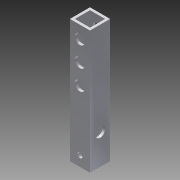
# Autodesk Inventor part: 1x1 vertical
Saved by Autodesk Inventor 2015 (Build 190159000, 159)
## iProperties
Created: 2015-01-27
Part Number: 1x1 vertical
Material: Aluminum 6061
Document SubType Name: Modeling
Designer: Admin
Density: 2.7 g/cm^3
Appearance: Aluminum - Flat
Author: Admin
Autodesk Inventor part; units mm, degrees
ref_plane "YZ Plane" through (0, 0, 0) normal (1, 0, 0) x (0, 1, 0)
ref_plane "XZ Plane" through (0, 0, 0) normal (0, 1, 0) x (-1, 0, 0)
ref_plane "XY Plane" through (0, 0, 0) normal (0, 0, 1) x (1, 0, 0)
sketch "Sketch1" plane through (0, 0, 0) normal (0, 1, 0) x (-1, 0, 0)
  line L0 (0, 0) -> (-25.4, 0)
  line L1 (-25.4, 0) -> (-25.4, -25.4)
  line L2 (-25.4, -25.4) -> (0, -25.4)
  line L3 (0, -25.4) -> (0, 0)
  line L4 (-3.175, -3.175) -> (-22.225, -3.175)
  line L5 (-22.225, -3.175) -> (-22.225, -22.225)
  line L6 (-22.225, -22.225) -> (-3.175, -22.225)
  line L7 (-3.175, -22.225) -> (-3.175, -3.175)
  dimension "d0" = 25.4
  dimension "d1" = 25.4
  dimension "d2" = 19.05
  dimension "d3" = 19.05
  dimension "d4" = 3.175
  dimension "d5" = 3.175
  constraints: 16 end point, 4 parallel, 2 horizontal, 2 perpendicular
  measures "d0" distance of L2.end L1.end
  measures "d1" distance of L1.end L0.end
  measures "d2" distance of L6.end L5.end
  measures "d3" distance of L5.end L4.end
  measures "d4" distance between parallel lines of L0 L4
  measures "d5" distance between parallel lines of L3 L7
extrude "Extrusion1" add sketch "Sketch1" along normal blind 155.575
sketch "Sketch2" plane through (0, 0, 0) normal (0, 0, 1) x (1, 0, 0)
  line L0 (0, 0) -> (25.4, 0) projected
  line L1 (0, 155.575) -> (25.4, 155.575) projected
  line L2 (0, 0) -> (0, 155.575) projected
  point P0 (12.7, 142.875)
  point P1 (12.7, 12.7)
  dimension "d8" = 12.7
  dimension "d9" = 12.7
  dimension "d10" = 12.7
  dimension "d11" = 12.7
  measures "d8" distance from line of L2 point (12.7, 142.875)
  measures "d9" distance from line of L1 point (12.7, 142.875)
  measures "d10" distance from line of L0 point (12.7, 12.7)
  measures "d11" distance from line of L2 point (12.7, 12.7)
hole "Hole1" at (12.7, 142.875, 0) at (12.7, 12.7, 0) direction (0, 0, -1) diameter 6.35 end through all
sketch "Sketch3" plane through (25.4, 0, 0) normal (1, 0, 0) x (0, 0, -1)
  line L0 (0, 0) -> (25.4, 0) projected
  line L1 (0, 0) -> (0, 155.575) projected
  point P0 (12.7, 38.1)
  dimension "d21" = 12.7
  dimension "d22" = 38.1
  measures "d21" distance from line of L1 point (12.7, 38.1)
  measures "d22" distance from line of L0 point (12.7, 38.1)
hole "Hole2" at (25.4, 38.1, -12.7) direction (-1, 0, 0) diameter 9.525 end through all
sketch "Sketch6" plane through (25.4, 0, 0) normal (1, 0, 0) x (0, 0, -1)
  circle A0 centre (12.7, 38.1) radius 4.7625 projected
  circle A1 centre (12.7, 38.1) radius 6.35
  dimension "d54" = 12.7
  constraints: 1 centre point, 1 coincident
  measures "d54" diameter of A1
extrude "Extrusion2" cut sketch "Sketch6" against normal blind 12.7
body "Solid1"
